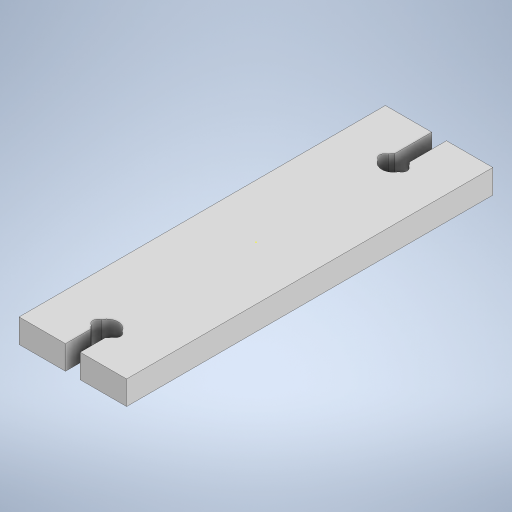
# Autodesk Inventor part: Male blade connector Plate
Saved by Autodesk Inventor 2023 (Build 270158000, 158)
## iProperties
Created: 2023-04-24
Part Number: Male blade connector Plate
Material: Generic
Document SubType Name: Modeling
Designer: mihal
Density: 1 g/cm^3
Appearance: Default
Author: mihal
Autodesk Inventor part; units mm, degrees
ref_plane "YZ Plane" through (0, 0, 0) normal (1, 0, 0) x (0, 1, 0)
ref_plane "XZ Plane" through (0, 0, 0) normal (0, 1, 0) x (-1, 0, 0)
ref_plane "XY Plane" through (0, 0, 0) normal (0, 0, 1) x (1, 0, 0)
sketch "Sketch1" plane through (0, 0, 0) normal (0, 1, 0) x (-1, 0, 0)
  line L0 (-13.5, 46) -> (13.5, 46)
  line L1 (13.5, 46) -> (13.5, -46)
  line L2 (13.5, -46) -> (-13.5, -46)
  line L3 (-13.5, -46) -> (-13.5, 46)
  line L4 (-13.5, 46) -> (13.5, -46) construction
  line L5 (13.5, 46) -> (-13.5, -46) construction
  point P0 (0, 0)
  dimension "d0" = 27
  dimension "d1" = 92
  constraints: 12 end point, 2 midpoint, 2 parallel, 1 horizontal, 1 perpendicular
  measures "d0" distance of L1.end L2.end
  measures "d1" distance of L0.end L1.end
extrude "Extrusion1" add sketch "Sketch1" along normal blind 6
sketch "Sketch2" plane through (0, 6, 0) normal (0, 1, 0) x (1, 0, 0)
  line L0 (13.5, 46) -> (-13.5, 46) projected
  line L1 (-13.5, 46) -> (-13.5, -46) projected
  line L2 (-13.5, -46) -> (13.5, -46) projected
  line L3 (13.5, -46) -> (13.5, 46) projected
  line L4 (0, -46) -> (0, -37.5) construction
  line L5 (0, 46) -> (0, 34.5) construction
  circle A0 centre (0, -37.5) radius 2.9
  circle A1 centre (0, 34.5) radius 2.9
  line L6 (0, 34.5) -> (1.85, 34.5) construction
  line L7 (0, 34.5) -> (-1.85, 34.5) construction
  line L8 (-1.85, 46) -> (-1.85, -46)
  line L9 (1.85, -46) -> (1.85, 46)
  ellipse E0 centre (0, 34.5) end of major axis (3.5, 34.5) minor radius 1.95
  line L10 (-13.5, 0) -> (13.5, 0) construction
  ellipse E1 centre (0, -37.5) end of major axis (3.5, -37.5) minor radius 1.95
  point P0 (0, 0)
  point P1 (-1.85, 36.7333)
  point P2 (1.85, 36.7333)
  point P3 (1.85, -39.7333)
  point P4 (-1.85, -39.7333)
  point P5 (2.5849, 35.8147)
  point P6 (2.5849, 33.1853)
  point P7 (-2.5849, 33.1853)
  point P8 (-2.5849, 35.8147)
  point P9 (-2.5849, -38.8147)
  point P10 (-2.5849, -36.1853)
  point P11 (2.5849, -36.1853)
  point P12 (2.5849, -38.8147)
  dimension "d12" = 1.95
  dimension "d13" = 3.5
  dimension "d14" = 1.95
  dimension "d15" = 3.5
  dimension "d4" = 8.5
  dimension "d5" = 11.5
  dimension "d6" = 5.8
  dimension "d7" = 5.8
  dimension "d8" = 1.85
  dimension "d9" = 1.85
  constraints: 14 end point, 6 point on line, 4 coincident, 4 midpoint, 2 centre point, 2 horizontal, 2 perpendicular, 2 vertical, 4 other
  measures "d4" distance of L4.start L4.end
  measures "d5" distance of L5.start L5.end
  measures "d6" diameter of A0
  measures "d7" diameter of A1
  measures "d8" distance of L6.start L6.end
  measures "d9" distance of L6.start L7.end
extrude "Extrusion2" cut sketch "Sketch2" against normal blind 6 contours L9 A1 L8 L0 | L9 E0 L8 A1 | A1 E0 L9 | L2 L8 A0 L9 | L8 E0 A1 | E0 A1 | A1 E0 L9 | L9 E0 L8 | L9 E1 A0 | A0 L8 E1 L9 | E0 L8 A1 | A1 E0 | E0 A1 L9 | L9 A1 L8 E0 | A0 E1 L8 | E1 L9 A0 | A0 E1 | E1 L8 L9 | E0 L8 A1 | E1 A0 | A0 E1 L8 | E1 L8 A0 L9 | L9 A0 E1 | A0 L8 E1
sketch "Sketch3" plane through (0, 6, 0) normal (0, 1, 0) x (1, 0, 0)
  point P0 (0, 0)
body "Solid1"
